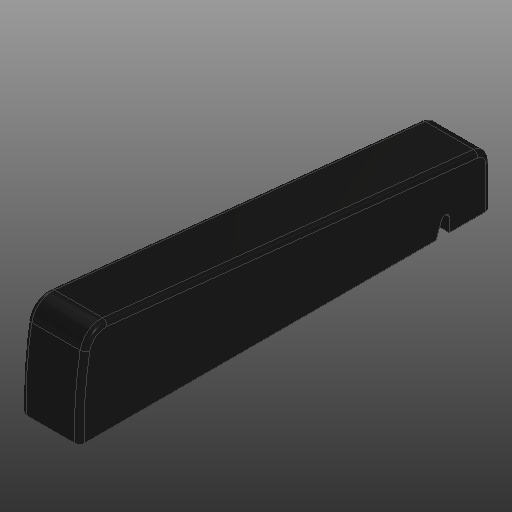
# Autodesk Inventor part: BlackKey0
Saved by Autodesk Inventor 2020 (Build 240168000, 168)
## iProperties
Created: 2019-12-01
Part Number: BlackKey0
Material: PLA Plastic (Black)
Document SubType Name: Modeling
Designer: Isaac Newcomb
Density: 1.06 g/cm^3
Appearance: 3D Printed - Black
Mass: 5.51831 g
Surface Area: 25.2749 cm^2
Volume: 5.20595 cm^3
Project: Ice Keys
hingeDepth: 2.000 mm
edgeSoftenRad: 0.700 mm
slotOffset: 1.047 mm
backWidth: 6.000 mm
hingeRad: 0.500 mm
hingeCutRad: 0.570 mm
slotHeadOffset: 1.000 mm
slotHeadHeight: 3.000 mm
slotHeadWidth: 6.000 mm
neckSlotWidth: 4.300 mm
blackKeyLength: 53.000 mm
cutoutWidth: 4.300 mm
keyHeight: 8.000 mm
headHeight: 3.000 mm
headOffset: 1.000 mm
d10: 1.600 mm
blackKeyWidth: 8.400 mm
keySpacing: 0.500 mm
Author: Isaac Newcomb
Autodesk Inventor part; units mm, degrees
ref_plane "YZ Plane" through (0, 0, 0) normal (1, 0, 0) x (0, 1, 0)
ref_plane "XZ Plane" through (0, 0, 0) normal (0, 1, 0) x (-1, 0, 0)
ref_plane "Slot Start Plane" through (0, 0, -1.617) normal (0, 0, 1) x (1, 0, 0)
sketch "Key Profile" plane through (0, 0, 0) normal (1, 0, 0) x (0, 1, 0)
  line L0 (-2, 2.4306) -> (0.5472, 1.5035)
  arc A0 (1.2099, -1.047) -> (0.5472, 1.5035) centre (0, 0) ccw
  line L1 (-2, 1.3345) -> (0.195, 0.5356)
  arc A1 (0, -0.57) -> (0.195, 0.5356) centre (0, 0) ccw
  line L2 (-2, 2.4306) -> (-2, -0.57)
  line L3 (0, 0) -> (-2, 0) construction
  line L4 (0, -0.57) -> (-2, -0.57)
  line L5 (1.2099, -1.047) -> (-0.1005, -0.57)
  line L6 (6, -4.7715) -> (12, 51.6236)
  line L7 (-2, 52.9623) -> (-2, 2.4306)
  arc A2 (12, 51.6236) -> (-2, 52.9623) centre (0, 0) ccw
  line L8 (-2, -0.57) -> (-2, -6.57)
  arc A3 (4, -6.57) -> (6, -4.7715) centre (4, -4.5587) ccw
  line L9 (-2, -6.57) -> (4, -6.57)
  dimension "hingeCutRad" = 0.57
  dimension "hingeDepth" = 2
  dimension "d10" = 1.6
  dimension "blackKeyLength" = 53
  dimension "blackKeyExtraHeight" = 6
  dimension "keyHeight" = 8
  dimension "d107" = 20
  dimension "d122" = 4
  dimension "slotOffset" = 1.047
  dimension "backWidth" = 6
  constraints: 21 end point, 9 point on circle, 6 tangent, 4 centre point, 3 coincident, 3 horizontal, 3 point on line, 2 parallel, 2 vertical, 1 collinear
  measures "hingeCutRad" radius of A1
  measures "hingeDepth" distance of L3.start L3.end
  measures "d10" radius of A0
  measures "blackKeyLength" radius of A2
  measures "blackKeyExtraHeight" horizontal distance of L6.start L6.end
  measures "keyHeight" distance from line of L6.start L7
  measures "d107" angle of L4 L1
  measures "d122" horizontal distance of A0.centre L9.end
  measures "slotOffset" vertical distance of L5.start point (0, 0)
  measures "backWidth" distance of L2.end L8.end
extrude "Key" add sketch "Key Profile" along normal mid plane 8.4 contours L7 A2 L6 A3 L9 L8 L4 L5 A0 L0 | L0 A0 L5 L4 A1 L1 L2
extrude "Protrusion Cutout" cut sketch "Key Profile" along normal mid plane 4.3 contours L0 A0 L5 L4 A1 L1 L2
fillet "Front Fillet" radius 3 1 edges at (0, 12, 51.6236)
sketch "Slot Sketch" plane through (0, 0, -1.617) normal (0, 0, 1) x (1, 0, 0)
  line L0 (2.15, -2) -> (2.15, 1)
  line L1 (3, 4) -> (-3, 4)
  line L2 (-2.15, 1) -> (-2.15, -2)
  line L3 (-2.15, -2) -> (2.15, -2)
  line L4 (0, -2) -> (0, 4) construction
  line L5 (-3, 4) -> (-3, 1)
  line L6 (-3, 1) -> (-2.15, 1)
  line L7 (2.15, 1) -> (3, 1)
  line L8 (3, 1) -> (3, 4)
  point P0 (0, 0)
  dimension "d109" = 2
  dimension "slotHeadOffset" = 1
  dimension "slotHeadHeight" = 3
  dimension "slotHeadWidth" = 6
  dimension "neckSlotWidth" = 4.3
  constraints: 18 end point, 4 perpendicular, 3 parallel, 2 midpoint, 2 point on line, 2 vertical
  measures "d109" distance from line of point (0, 0) L3
  measures "slotHeadOffset" distance from line of L6 point (0, 0)
  measures "slotHeadHeight" distance of L1.end L5.end
  measures "slotHeadWidth" distance of L1.start L1.end
  measures "neckSlotWidth" distance of L2.end L0.start
extrude "Slot" cut sketch "Slot Sketch" against normal through all
fillet "Edge Softening" radius 0.7 10 edges at (4.2, 11.1265, 51.035) (4.2, 3.6469, 52.8744) (4.2, 5.3449, -6.0542) (4.2, 1, -6.57) (4.2, 8.8559, 22.0717) (-4.2, 5.3449, -6.0542) (-4.2, 1, -6.57) (-4.2, 11.1265, 51.035) (-4.2, 3.6469, 52.8744) (-4.2, 8.8559, 22.0717)
equation "\"headHeight\" = 3"
equation "\"headOffset\" = 1"
equation "\"keySpacing\" = 0.5"
body "Solid1"
